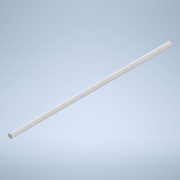
# Autodesk Inventor part: spirale
Saved by Autodesk Inventor 2022 (Build 260153000, 153)
## iProperties
Created: 2022-01-15
Part Number: spirale
Material: Generic
Document SubType Name: Modeling
Designer: simon
Density: 1 g/cm^3
Appearance: Default
Author: simon
Autodesk Inventor part; units mm, degrees
ref_plane "YZ Plane" through (0, 0, 0) normal (1, 0, 0) x (0, 1, 0)
ref_plane "XZ Plane" through (0, 0, 0) normal (0, 1, 0) x (-1, 0, 0)
ref_plane "XY Plane" through (0, 0, 0) normal (0, 0, 1) x (1, 0, 0)
sketch "Sketch1" plane through (0, 0, 0) normal (0, 0, 1) x (1, 0, 0)
  circle A0 centre (0, 0) radius 4.05 projected
  circle A1 centre (0, 0) radius 7.5 projected
  circle A2 centre (0, 0) radius 4.05 projected
  circle A3 centre (0, 0) radius 4
  dimension "d0" = 8
  constraints: 1 centre point, 1 coincident
  measures "d0" diameter of A3
extrude "Extrusion1" add sketch "Sketch1" along normal blind 100 contours A3
sketch "Sketch2" plane through (0, 0, 100) normal (0, 0, 1) x (1, 0, 0)
  circle A0 centre (0, 0) radius 4 projected
  line L0 (-1.5, 4) -> (-1.5, -4)
  line L1 (-1.5, -4) -> (1.5, -4)
  line L2 (1.5, -4) -> (1.5, 4)
  line L3 (1.5, 4) -> (-1.5, 4)
  line L4 (-1.5, 4) -> (1.5, -4) construction
  line L5 (-1.5, -4) -> (1.5, 4) construction
  point P0 (-1.5, -3.7081)
  point P1 (-1.5, 3.7081)
  point P2 (1.5, 3.7081)
  point P3 (1.5, -3.7081)
  dimension "d3" = 3
  constraints: 12 end point, 2 midpoint, 2 parallel, 1 perpendicular, 1 vertical
  measures "d3" distance of L1.end L0.end
extrude "Extrusion2" add sketch "Sketch2" along normal blind 50 contours A0 L2 | L0 A0
body "Solid1"
